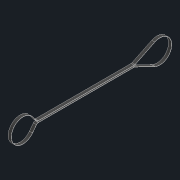
# Autodesk Inventor part: scara-belt1
Saved by Autodesk Inventor 2022 (Build 260153000, 153)
## iProperties
Created: 2021-07-18
Part Number: scara-belt1
Material: ゴム
Document SubType Name: Modeling
Designer: yuta0
Density: 0.93 g/cm^3
Appearance: ゴム - 黒
Mass: 8.55769 g
Surface Area: 248.449 cm^2
Volume: 9.20182 cm^3
Description: ミスミ
購入先: ミスミ
在庫数: 0.0
Author: yuta0
Autodesk Inventor part; units mm, degrees
ref_plane "YZ Plane" through (0, 0, 0) normal (1, 0, 0) x (0, 1, 0)
ref_plane "XZ Plane" through (0, 0, 0) normal (0, 1, 0) x (-1, 0, 0)
ref_plane "XY Plane" through (0, 0, 0) normal (0, 0, 1) x (1, 0, 0)
sketch "スケッチ1" plane through (0, 0, 0) normal (1, 0, 0) x (0, 1, 0)
  arc A0 (23.0723, -31.0387) -> (-23.0723, -31.0387) centre (0, 0) ccw
  arc A1 (-34.7971, -433.1214) -> (34.7971, -433.1214) centre (0, -450) ccw
  arc A2 (-2.581, -50) -> (-5.574, -44.0458) centre (-10, -50) ccw
  line L0 (-5.574, -44.0458) -> (-23.0723, -31.0387)
  line L1 (23.0723, -31.0387) -> (5.574, -44.0458)
  line L2 (34.7971, -433.1214) -> (3.3248, -368.2378)
  line L3 (-34.7971, -433.1214) -> (-3.3248, -368.2378)
  arc A3 (5.574, -44.0458) -> (2.581, -50) centre (10, -50) ccw
  arc A4 (2.581, -365) -> (3.3248, -368.2378) centre (10, -365) ccw
  arc A5 (-3.3248, -368.2378) -> (-2.581, -365) centre (-10, -365) ccw
  line L4 (-2.581, -50) -> (-2.581, -365)
  line L5 (2.581, -365) -> (2.581, -50)
  line L6 (5.824, -44.3821) -> (23.3222, -31.3749)
  arc A6 (23.3222, -31.3749) -> (-23.3222, -31.3749) centre (0, 0) ccw
  line L7 (-23.3222, -31.3749) -> (-5.824, -44.3821)
  arc A7 (-3, -50) -> (-5.824, -44.3821) centre (-10, -50) ccw
  line L8 (-3, -50) -> (-3, -365)
  arc A8 (-3.7018, -368.055) -> (-3, -365) centre (-10, -365) ccw
  line L9 (-3.7018, -368.055) -> (-35.1741, -432.9385)
  arc A9 (-35.1741, -432.9385) -> (35.1741, -432.9385) centre (0, -450) ccw
  line L10 (35.1741, -432.9385) -> (3.7018, -368.055)
  arc A10 (3, -365) -> (3.7018, -368.055) centre (10, -365) ccw
  line L11 (3, -365) -> (3, -50)
  arc A11 (5.824, -44.3821) -> (3, -50) centre (10, -50) ccw
  arc A12 (5.3467, -43.74) -> (2.2, -50) centre (10, -50) ccw
  line L12 (5.3467, -43.74) -> (22.845, -30.7329)
  arc A13 (22.845, -30.7329) -> (-22.845, -30.7329) centre (0, 0) ccw
  line L13 (-22.845, -30.7329) -> (-5.3467, -43.74)
  arc A14 (-2.2, -50) -> (-5.3467, -43.74) centre (-10, -50) ccw
  line L14 (-2.2, -50) -> (-2.2, -365)
  arc A15 (-2.982, -368.4041) -> (-2.2, -365) centre (-10, -365) ccw
  line L15 (-2.982, -368.4041) -> (-34.4543, -433.2876)
  arc A16 (-34.4543, -433.2876) -> (34.4543, -433.2876) centre (0, -450) ccw
  line L16 (34.4543, -433.2876) -> (2.982, -368.4041)
  arc A17 (2.2, -365) -> (2.982, -368.4041) centre (10, -365) ccw
  line L17 (2.2, -365) -> (2.2, -50)
  dimension "d0" = 77.3493
  dimension "d1" = 77.3493
  dimension "d2" = 450
  dimension "d39" = 0.419
  dimension "d40" = 0.8
  dimension "d41" = 7
  dimension "d42" = 7
  dimension "d43" = 7
  dimension "d44" = 7
  dimension "d45" = 10
  dimension "d46" = 10
  dimension "d47" = 85
  dimension "d48" = 50
  constraints: 36 end point, 36 point on circle, 18 centre point, 12 tangent, 3 vertical alignment, 2 horizontal alignment, 1 coincident, 22 other
  measures "d0" diameter of A0
  measures "d1" diameter of A1
  measures "d2" distance of A0.centre A1.centre
  measures "d39" distance between parallel lines of L11 L5
  measures "d40" distance between parallel lines of L11 L17
  measures "d41" radius of A11
  measures "d42" radius of A7
  measures "d43" radius of A10
  measures "d44" radius of A8
  measures "d45" horizontal distance of point (0, 0) A3.centre
  measures "d46" horizontal distance of point (0, 0) A2.centre
  measures "d47" vertical distance of A1.centre A4.centre
  measures "d48" vertical distance of point (0, 0) A3.centre
extrude "押し出し1" add sketch "スケッチ1" along normal mid plane 10 contours L1 A3 L5 A4 L2 A1 L3 A5 L4 A2 L0 A0 | A11 L11 A10 L10 A9 L9 A8 L8 A7 L7 A6 L6
equation "\"d0\" = d1"
equation "\"d41\" = d43"
equation "\"d43\" = d44"
equation "\"d44\" = d42"
equation "\"d46\" = d45"
